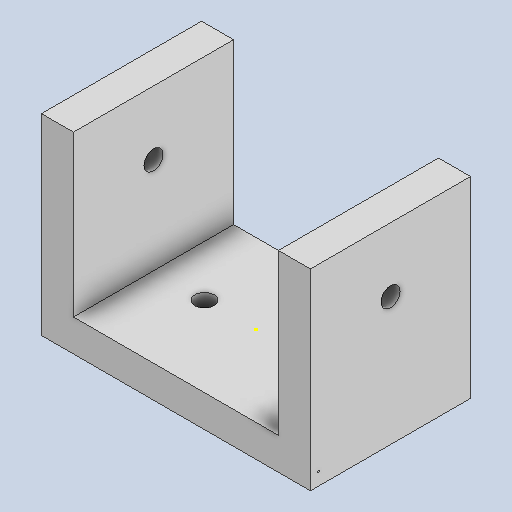
# Autodesk Inventor part: clamp
Saved by Autodesk Inventor 2023 (Build 270158000, 158)
## iProperties
Created: 2022-06-14
Part Number: clamp
Material: Generic
Document SubType Name: Modeling
Designer: chait
Density: 1 g/cm^3
Appearance: Default
Author: chait
Autodesk Inventor part; units mm, degrees
ref_plane "YZ Plane" through (0, 0, 0) normal (1, 0, 0) x (0, 1, 0)
ref_plane "XZ Plane" through (0, 0, 0) normal (0, 1, 0) x (-1, 0, 0)
ref_plane "XY Plane" through (0, 0, 0) normal (0, 0, 1) x (1, 0, 0)
sketch "Sketch1" plane through (0, 0, 0) normal (0, 1, 0) x (-1, 0, 0)
  line L0 (21, 12.5) -> (-21, 12.5)
  line L1 (-21, 12.5) -> (-21, -12.5)
  line L2 (-21, -12.5) -> (21, -12.5)
  line L3 (21, -12.5) -> (21, 12.5)
  line L4 (21, 12.5) -> (-21, -12.5) construction
  line L5 (-21, 12.5) -> (21, -12.5) construction
  point P0 (0, 0)
  dimension "d0" = 42
  dimension "d1" = 25
  constraints: 12 end point, 2 midpoint, 2 parallel, 1 horizontal, 1 perpendicular
  measures "d0" distance of L2.end L1.end
  measures "d1" distance of L1.end L0.end
extrude "Extrusion1" add sketch "Sketch1" along normal blind 5
sketch "Sketch5" plane through (-21, 0, -12.5) normal (-1, 0, 0) x (0, 0, 1)
  point P0 (12.5, 0)
sketch "Sketch6" plane through (21, 0, 12.5) normal (1, 0, 0) x (0, 0, -1)
  circle A0 centre (1.25, 2.0074) radius 0.15
  point P0 (12.5, 0)
  dimension "d11" = 0.3
  constraints: 1 centre point
  measures "d11" diameter of A0
extrude "Extrusion5" cut sketch "Sketch6" against normal blind 10
sketch "Sketch8" plane through (0, 5, 0) normal (0, 1, 0) x (1, 0, 0)
  line L0 (21, 12.5) -> (-21, 12.5) projected
  line L1 (-21, -12.5) -> (21, -12.5) projected
  line L2 (-21, 12.5) -> (-16, 12.5)
  line L3 (-16, 12.5) -> (-16, -12.5)
  line L4 (-16, -12.5) -> (-21, -12.5)
  line L5 (-21, -12.5) -> (-21, 12.5)
  point P0 (0, 0)
  dimension "d14" = 5
  constraints: 8 end point, 2 parallel, 1 horizontal, 1 perpendicular, 1 point on line
  measures "d14" distance of L3.end L4.end
extrude "Extrusion6" add sketch "Sketch8" along normal blind 25
sketch "Sketch9" plane through (0, 5, 0) normal (0, 1, 0) x (1, 0, 0)
  line L0 (21, 12.5) -> (-21, 12.5) projected
  line L1 (-21, -12.5) -> (21, -12.5) projected
  line L2 (21, 12.5) -> (16, 12.5)
  line L3 (16, 12.5) -> (16, -12.5)
  line L4 (16, -12.5) -> (21, -12.5)
  line L5 (21, -12.5) -> (21, 12.5)
  point P0 (0, 0)
  point P1 (16, 12.5)
  dimension "d17" = 5
  constraints: 8 end point, 2 parallel, 1 horizontal, 1 perpendicular, 1 point on line
  measures "d17" distance of L4.end L3.end
extrude "Extrusion7" add sketch "Sketch9" along normal blind 25
sketch "Sketch10" plane through (21, 0, 12.5) normal (1, 0, 0) x (0, 0, -1)
  circle A0 centre (12.5, 19.9992) radius 1.5
  point P0 (12.5, 0)
  dimension "d20" = 3
  constraints: 1 centre point
  measures "d20" diameter of A0
extrude "Extrusion8" cut sketch "Sketch10" against normal blind 100
sketch "Sketch11" plane through (0, 5, 0) normal (0, 1, 0) x (1, 0, 0)
  point P0 (0, 0)
sketch "Sketch12" plane through (0, 5, 0) normal (0, 1, 0) x (1, 0, 0)
  circle A0 centre (-8.051, 0) radius 1.5
  circle A1 centre (8.051, 0) radius 1.5
  point P0 (0, 0)
  dimension "d23" = 3
  dimension "d24" = 3
  constraints: 2 centre point
  measures "d23" diameter of A0
  measures "d24" diameter of A1
extrude "Extrusion9" cut sketch "Sketch12" against normal blind 10
body "Solid1"
